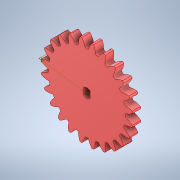
# Autodesk Inventor part: Engranaje B
Saved by Autodesk Inventor 2020.3 (Build 243373000, 373)
## iProperties
Created: 2020-07-27
Part Number: Engranaje B
Material: ABS Plastic
Document SubType Name: Modeling
Designer: juanp
Density: 1.06 g/cm^3
Appearance: Smooth - White
Author: juanp
Autodesk Inventor part; units mm, degrees
ref_plane "YZ Plane" through (0, 0, 0) normal (1, 0, 0) x (0, 1, 0)
ref_plane "XZ Plane" through (0, 0, 0) normal (0, 1, 0) x (-1, 0, 0)
ref_plane "XY Plane" through (0, 0, 0) normal (0, 0, 1) x (1, 0, 0)
sketch "Sketch1" plane through (0, 0, 0) normal (0, 0, 1) x (1, 0, 0)
  spline S0 degree 3 poles (-3.0247, 27.2426) (-2.9533, 27.1511) (-2.8105, 26.9681) (-2.6049, 26.6871) (-2.4062, 26.4011) (-2.2156, 26.1098) (-2.0333, 25.8131) (-1.8602, 25.511) (-1.697, 25.2034) (-1.5447, 24.8902) (-1.4044, 24.5715) (-1.2782, 24.247) (-1.167, 23.9167) (-1.0941, 23.6364) (-1.0491, 23.4373) (-0.9989, 23.3323) (-0.9533, 23.258) (-0.8982, 23.1903) (-0.8348, 23.1303) (-0.764, 23.0793) (-0.6878, 23.0369) (-0.6066, 23.0051) (-0.522, 22.9837) (-0.4352, 22.974) (-0.261, 22.9763) (0, 22.9798) (0.261, 22.9763) (0.4352, 22.974) (0.522, 22.9837) (0.6066, 23.0051) (0.6878, 23.0369) (0.764, 23.0793) (0.8348, 23.1303) (0.8982, 23.1903) (0.9533, 23.258) (0.9989, 23.3323) (1.0491, 23.4373) (1.0941, 23.6364) (1.167, 23.9167) (1.2782, 24.247) (1.4044, 24.5715) (1.5447, 24.8902) (1.697, 25.2034) (1.8602, 25.511) (2.0333, 25.8131) (2.2156, 26.1098) (2.4062, 26.4011) (2.6049, 26.6871) (2.8105, 26.9681) (2.9533, 27.1511) (3.0247, 27.2426) knots 0 0 0 0 0.034815 0.06963 0.104445 0.13926 0.174075 0.20889 0.243705 0.278519 0.313332 0.348146 0.382957 0.417766 0.435155 0.443855 0.452557 0.461257 0.469958 0.478659 0.487361 0.496063 0.504763 0.513463 0.522168 0.556982 0.591795 0.600501 0.6092 0.6179 0.626603 0.635304 0.644005 0.652706 0.661407 0.670108 0.678808 0.696198 0.731006 0.765818 0.800631 0.835445 0.870259 0.905073 0.939888 0.974703 1.009518 1.044333 1.079148 1.113963 1.113963 1.113963 1.113963
  circle A0 centre (0, 0) radius 22.9782 construction
  circle A1 centre (0, 0) radius 23.2355 construction
  circle A2 centre (0, 0) radius 24 construction
  circle A3 centre (0, 0) radius 27.41
  point P0 (-2.8119, 26.967)
  point P1 (-2.606, 26.6863)
  point P2 (-2.4076, 26.4002)
  point P3 (-2.217, 26.1089)
  point P4 (-2.0348, 25.8122)
  point P5 (-1.8619, 25.51)
  point P6 (-1.6988, 25.2024)
  point P7 (-1.5467, 24.8893)
  point P8 (-1.4068, 24.5705)
  point P9 (-1.2807, 24.246)
  point P10 (-1.171, 23.9156)
  point P11 (-1.0818, 23.5792)
  point P12 (-1.0345, 23.4118)
  point P13 (-0.9975, 23.3331)
  point P14 (-0.9517, 23.2591)
  point P15 (-0.8968, 23.1916)
  point P16 (-0.8336, 23.1318)
  point P17 (-0.7631, 23.0808)
  point P18 (-0.687, 23.0387)
  point P19 (-0.606, 23.0068)
  point P20 (-0.5216, 22.9856)
  point P21 (-0.4352, 22.9758)
  point P22 (-0.3481, 22.9751)
  point P23 (0, 22.9782)
  point P24 (0.3481, 22.9751)
  point P25 (0.4352, 22.9758)
  point P26 (0.5216, 22.9856)
  point P27 (0.606, 23.0068)
  point P28 (0.687, 23.0387)
  point P29 (0.7631, 23.0808)
  point P30 (0.8336, 23.1318)
  point P31 (0.8968, 23.1916)
  point P32 (0.9517, 23.2591)
  point P33 (0.9975, 23.3331)
  point P34 (1.0345, 23.4118)
  point P35 (1.0818, 23.5792)
  point P36 (1.171, 23.9156)
  point P37 (1.2807, 24.246)
  point P38 (1.4068, 24.5705)
  point P39 (1.5467, 24.8893)
  point P40 (1.6988, 25.2024)
  point P41 (1.8619, 25.51)
  point P42 (2.0348, 25.8122)
  point P43 (2.217, 26.1089)
  point P44 (2.4076, 26.4002)
  point P45 (2.606, 26.6863)
  point P46 (2.8119, 26.967)
  constraints: 4 centre point, 2 point on circle, 103 other
extrude "Extrusion1" add sketch "Sketch1" against normal blind 5
extrude "Extrusion2" cut sketch "Sketch1" against normal through all contours A3 S0 picked at (0.4132, 25.9217)
pattern_circular "Circular Pattern1" count 24 over 360 about axis through (0, 0, 0) along (0, 0, -1) of "Extrusion2"
sketch "Sketch3" plane through (0, 0, 0) normal (0, 0, 1) x (1, 0, 0)
  arc A0 (-27.0972, 4.1293) -> (-27.2426, 3.0247) centre (0, 0) ccw projected
  line L0 (-27.2426, 3.0247) -> (-27.0972, 4.1293)
  point P0 (-27.1699, 3.577)
  constraints: 2 end point, 1 midpoint
sketch "Sketch4" plane through (0, 0, -5) normal (0, 0, -1) x (-1, 0, 0)
  arc A0 (27.2426, 3.0247) -> (27.0972, 4.1293) centre (0, 0) ccw projected
  line L0 (27.2426, 3.0247) -> (27.0972, 4.1293)
  point P0 (27.1699, 3.577)
  constraints: 2 end point, 1 midpoint
ref_plane "Work Plane1" through (-27.1699, 3.577, -5) normal (0.1305262, 0.9914449, 0) x (0, 0, 1)
sketch "Sketch5" plane through (0, 0, -5) normal (0, 0, -1) x (-1, 0, 0)
  arc A0 (-1.9, -1.9881) -> (1.9, -1.9881) centre (0, 0) ccw
  line L0 (-1.9, 1.9881) -> (1.9, 1.9881) construction
  line L1 (1.9, 1.9881) -> (1.9, -1.9881)
  line L2 (1.9, -1.9881) -> (-1.9, -1.9881) construction
  line L3 (-1.9, -1.9881) -> (-1.9, 1.9881)
  arc A1 (-1.9, 1.9881) -> (-1.9, -1.9881) centre (0, 0) ccw construction
  arc A2 (1.9, -1.9881) -> (1.9, 1.9881) centre (0, 0) ccw construction
  arc A3 (1.9, 1.9881) -> (-1.9, 1.9881) centre (0, 0) ccw
  dimension "d7" = 5.5
  dimension "d9" = 3.8
  constraints: 9 point on circle, 8 end point, 4 centre point, 2 parallel, 1 coincident, 1 horizontal, 1 perpendicular
  measures "d7" diameter of A0
  measures "d9" distance between parallel lines of L1 L3
extrude "Extrusion3" cut sketch "Sketch5" against normal through all
equation "\"d0\" = FaceWidth"
equation "\"Module\" = 2"
equation "\"PressureAngle\" = 14.5deg"
equation "\"UnitProfileClearance\" = 0.25"
equation "\"UnitRoundRadius\" = 0.3335"
equation "\"HeadDiameter\" = 54.82"
equation "\"RootDiameter\" = 45.95647"
equation "\"BaseDiameter\" = 46.47109"
equation "\"PitchDiameter\" = 48"
equation "\"FaceWidth\" = 5"
equation "\"HelixAngle\" = 0"
equation "\"UnitCorrection\" = 0.838966"
equation "\"UnitAddendumModification\" = 0.133966"
equation "\"CircularPitch\" = 6.283185"
equation "\"UnitBacklashShift\" = -0.099848"
equation "\"TotalToolShift\" = 1.47824"
equation "\"IsInternal\" = 0"
body "Solid1"
